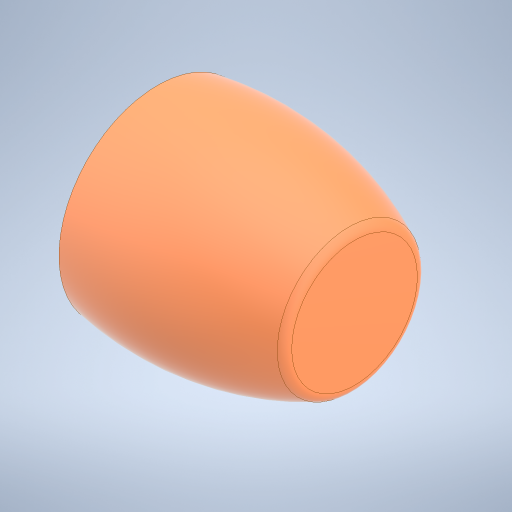
# Autodesk Inventor part: Bucket
Saved by Autodesk Inventor 2024.2 (Build 282272000, 272)
## iProperties
Created: 2024-01-18
Part Number: Bucket
Material: LCP Plastic
Document SubType Name: Modeling
Designer: airso
Density: 1.626 g/cm^3
Appearance: Smooth - White
Author: airso
Autodesk Inventor part; units mm, degrees
ref_plane "YZ Plane" through (0, 0, 0) normal (1, 0, 0) x (0, 1, 0)
ref_plane "XZ Plane" through (0, 0, 0) normal (0, 1, 0) x (-1, 0, 0)
ref_plane "XY Plane" through (0, 0, 0) normal (0, 0, 1) x (1, 0, 0)
sketch "Sketch1" plane through (0, 0, 0) normal (0, 1, 0) x (-1, 0, 0)
  line L0 (0, 0) -> (0, -254)
  line L1 (0, 0) -> (-508, 0)
  line L2 (-508, 0) -> (-508, -162.0489)
  arc A0 (-493.6643, -184.9125) -> (0, -254) centre (-139.6069, 546.7208) ccw
  arc A1 (-508, -162.0489) -> (-493.6643, -184.9125) centre (-482.6, -162.0489) ccw
  line L3 (-495.3, -12.7) -> (-495.3, -162.0489)
  arc A2 (-495.3, -162.0489) -> (-488.1321, -173.4807) centre (-482.6, -162.0489) ccw
  arc A3 (-488.1321, -173.4807) -> (-12.7, -243.2505) centre (-139.6069, 546.7208) ccw
  line L4 (-495.3, -12.7) -> (-495.3, 0)
  line L5 (-12.7, -243.2505) -> (0, -243.2505)
  point P0 (-508, -177.8)
  dimension "d0" = 254
  dimension "d1" = 508
  dimension "d2" = 177.8
  dimension "d3" = 25.4
  dimension "d4" = 812.8
  dimension "d5" = 12.7
  dimension "d6" = 12.7
  constraints: 12 end point, 9 point on circle, 4 centre point, 3 point on line, 2 perpendicular, 2 tangent, 2 vertical, 1 horizontal, 2 other
  measures "d0" distance of L0.start L0.end
  measures "d1" distance of L0.start L1.end
  measures "d2" distance of L1.end point (-508, -177.8)
  measures "d3" radius of A1
  measures "d4" radius of A0
  measures "d5" radial gap between concentric circles of A0 A3
  measures "d6" distance of L5.start L5.end
revolve "Revolution1" add sketch "Sketch1" angle 360 about axis through (0, 0, 0) along (1, 0, 0) contours L0 A0 A1 L2 L1 L4 L3 A2 A3 L5
body "Solid1"
